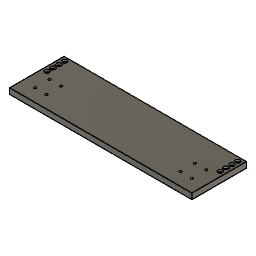
riser base plate (Autodesk Fusion 360 design; units mm, degrees)
Autodesk Fusion 360 part; units mm, degrees
sketch "Sketch1" plane through (0, 0, 0) normal (0, 0, 1) x (1, 0, 0)
  line L0 (0, 0) -> (320, 0)
  line L1 (320, 0) -> (320, 100)
  line L2 (320, 100) -> (0, 100)
  line L3 (0, 100) -> (0, 0)
  dimension "d1" = 320
  dimension "d2" = 100
  constraint horizontal L0
  constraint vertical L1
  constraint horizontal L2
  constraint vertical L3
  constraint coincident L0.start L3.end
  measures "d1" distance of L0.start L0.end
  measures "d2" distance of L0.start L2.end
extrude "Extrude1" add sketch "Sketch1" along normal blind 10
sketch "Sketch2" plane through (0, 0, 10) normal (0, 0, 1) x (-1, 0, 0)
  line L0 (0, -100) -> (0, 0)
  line L1 (0, 0) -> (-320, 0)
  line L2 (-320, 0) -> (-320, -100)
  line L3 (-320, -100) -> (0, -100)
  circle A0 centre (-11, -90) radius 2.25
  circle A1 centre (-309, -90) radius 2.25
  circle A2 centre (-11, -80) radius 2.25
  circle A3 centre (-309, -80) radius 2.25
  circle A4 centre (-11, -70) radius 2.25
  circle A5 centre (-11, -60) radius 2.25
  circle A6 centre (-309, -70) radius 2.25
  circle A7 centre (-309, -60) radius 2.25
  dimension "d5" = 4.5
  dimension "d6" = 4.5
  dimension "d7" = 298
  dimension "d8" = 11
  dimension "d9" = 10
  dimension "d10" = 4.5
  dimension "d11" = 4.5
  dimension "d13" = 4.5
  dimension "d14" = 4.5
  dimension "d16" = 4.5
  dimension "d17" = 4.5
  measures "d5" diameter of A0
  measures "d6" diameter of A1
  measures "d7" distance of A0.centre A1.centre
  measures "d8" distance of L0 A0.centre
  measures "d9" distance of L3 A0.centre
  measures "d10" diameter of A2
  measures "d11" diameter of A3
  measures "d13" diameter of A4
  measures "d14" diameter of A6
  measures "d16" diameter of A5
  measures "d17" diameter of A7
extrude "Extrude2" cut sketch "Sketch2" against normal blind 30 contours A0 | A1 | A2 | A3 | A4 | A5 | A6 | A7
sketch "Sketch3" plane through (0, 0, 10) normal (0, 0, 1) x (-1, 0, 0)
  circle A0 centre (-309, -80) radius 2.25
  circle A1 centre (-11, -80) radius 2.25
  circle A2 centre (-11, -70) radius 2.25
  circle A3 centre (-309, -70) radius 2.25
  circle A4 centre (-309, -90) radius 2.25
  circle A5 centre (-11, -90) radius 2.25
  circle A6 centre (-11, -60) radius 2.25
  circle A7 centre (-309, -60) radius 2.25
  line L0 (0, -100) -> (0, 0)
  line L1 (0, 0) -> (-320, 0)
  line L2 (-320, 0) -> (-320, -100)
  line L3 (-320, -100) -> (0, -100)
  circle A8 centre (-11, -90) radius 4
  dimension "d23" = 8
  constraint concentric A5 A8
  measures "d23" diameter of A8
extrude "Extrude3" cut sketch "Sketch3" against normal blind 3.5 contours A8
pattern_linear "R-Pattern1" count 4 spacing 10 along (0, -1, 0) count 2 spacing 298 along (1, 0, 0) of "Extrude3"
sketch "Sketch4" plane through (0, 0, 10) normal (0, 0, 1) x (-1, 0, 0)
  circle A0 centre (-309, -60) radius 4
  circle A1 centre (-309, -70) radius 4
  circle A2 centre (-309, -80) radius 4
  circle A3 centre (-309, -90) radius 4
  circle A4 centre (-11, -60) radius 4
  circle A5 centre (-11, -70) radius 4
  circle A6 centre (-11, -80) radius 4
  circle A7 centre (-11, -90) radius 4
  line L0 (0, -100) -> (0, 0)
  line L1 (0, 0) -> (-320, 0)
  line L2 (-320, 0) -> (-320, -100)
  line L3 (-320, -100) -> (0, -100)
  line L4 (-317, -3) -> (-3, -3)
  line L5 (-3, -3) -> (-3, -97)
  line L6 (-3, -97) -> (-317, -97)
  line L7 (-317, -97) -> (-317, -3)
  constraint horizontal L4
  constraint vertical L5
  constraint horizontal L6
  constraint vertical L7
extrude "Extrude4" add sketch "Sketch4" along normal blind 5 contours L0 L1 L2 L3
sketch "Sketch5" plane through (0, 0, 10) normal (0, 0, 1) x (-1, 0, 0)
  line L0 (-3, -97) -> (-3, -3)
  line L1 (-3, -3) -> (-317, -3)
  line L2 (-317, -3) -> (-317, -97)
  line L3 (-317, -97) -> (-3, -97)
  circle A0 centre (-309, -60) radius 4
  circle A1 centre (-309, -70) radius 4
  circle A2 centre (-309, -80) radius 4
  circle A3 centre (-309, -90) radius 4
  circle A4 centre (-11, -60) radius 4
  circle A5 centre (-11, -70) radius 4
  circle A6 centre (-11, -80) radius 4
  circle A7 centre (-11, -90) radius 4
  circle A8 centre (-25, -50) radius 2.075
  circle A9 centre (-25, -25) radius 2.075
  circle A10 centre (-295, -50) radius 2.075
  circle A11 centre (-295, -25) radius 2.075
  dimension "d32" = 4.15
  dimension "d33" = 4.15
  dimension "d34" = 4.15
  dimension "d35" = 4.15
  measures "d32" diameter of A8
  measures "d33" diameter of A9
  measures "d34" diameter of A10
  measures "d35" diameter of A11
extrude "Extrude5" add sketch "Sketch5" along normal blind 3 contours A8 | A9 | A10 | A11
sketch "Sketch6" plane through (0, 0, 10) normal (0, 0, 1) x (-1, 0, 0)
  circle A0 centre (-295, -25) radius 2.075
  circle A1 centre (-25, -50) radius 2.075
  circle A2 centre (-295, -50) radius 2.075
  circle A3 centre (-25, -25) radius 2.075
  line L0 (-3, -97) -> (-3, -3)
  line L1 (-3, -3) -> (-317, -3)
  line L2 (-317, -3) -> (-317, -97)
  line L3 (-317, -97) -> (-3, -97)
  circle A4 centre (-309, -60) radius 4
  circle A5 centre (-309, -70) radius 4
  circle A6 centre (-309, -80) radius 4
  circle A7 centre (-309, -90) radius 4
  circle A8 centre (-11, -60) radius 4
  circle A9 centre (-11, -70) radius 4
  circle A10 centre (-11, -80) radius 4
  circle A11 centre (-11, -90) radius 4
  circle A12 centre (-45, -50) radius 2.075
  circle A13 centre (-45, -25) radius 2.075
  circle A14 centre (-275, -50) radius 2.075
  circle A15 centre (-275, -25) radius 2.075
  dimension "d38" = 4.15
  dimension "d39" = 4.15
  dimension "d40" = 4.15
  dimension "d41" = 4.15
  measures "d38" diameter of A12
  measures "d39" diameter of A13
  measures "d40" diameter of A14
  measures "d41" diameter of A15
extrude "Extrude6" cut sketch "Sketch6" against normal blind 3 contours A12 | A13 | A14 | A15
extrude "Extrude7" cut 1 faces at (212.3333, 1, 15) along direction (0, 0, -1) blind 15
extrude "Extrude8" cut 4 faces at (24.3391, 50.0023, 13) (25.1539, 24.4763, 13) (295.5715, 25.5958, 13) (294.4285, 49.4042, 13) along direction (0, 0, -1) blind 6
